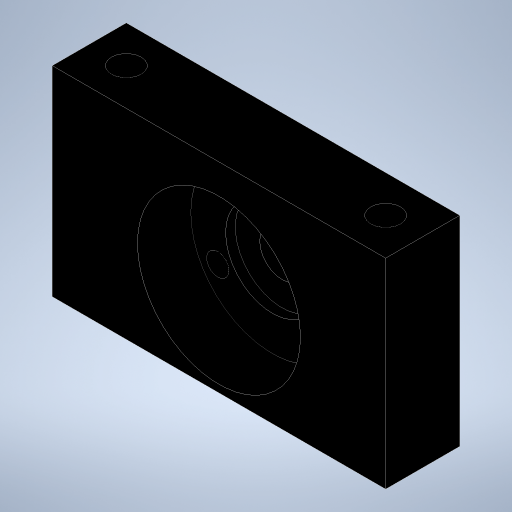
# Autodesk Inventor part: MotorBracket
Saved by Autodesk Inventor 2024 (Build 280153000, 153)
## iProperties
Created: 2023-02-23
Part Number: MotorBracket
Material: Generic
Document SubType Name: Modeling
Designer: Elias Braun
Density: 1 g/cm^3
Appearance: Default
Author: Elias Braun
Autodesk Inventor part; units mm, degrees
ref_plane "YZ Plane" through (0, 0, 0) normal (1, 0, 0) x (0, 1, 0)
ref_plane "XZ Plane" through (0, 0, 0) normal (0, 1, 0) x (-1, 0, 0)
ref_plane "XY Plane" through (0, 0, 0) normal (0, 0, 1) x (1, 0, 0)
sketch "Sketch1" plane through (0, 0, 0) normal (0, 1, 0) x (-1, 0, 0)
  line L0 (22.5, 5) -> (-22.5, 5)
  line L1 (-22.5, 5) -> (-22.5, -5)
  line L2 (-22.5, -5) -> (22.5, -5)
  line L3 (22.5, -5) -> (22.5, 5)
  line L4 (22.5, 5) -> (-22.5, -5) construction
  line L5 (-22.5, 5) -> (22.5, -5) construction
  line L6 (0, 0) -> (17.5, 0) construction
  line L7 (0, 0) -> (-17.5, 0) construction
  circle A0 centre (17.5, 0) radius 2
  circle A1 centre (-17.5, 0) radius 2
  line L8 (22.5, 5) -> (17.5, 5)
  line L9 (17.5, 5) -> (17.5, 0) construction
  dimension "d0" = 45
  dimension "d1" = 10
  dimension "d2" = 17.5
  dimension "d3" = 17.5
  dimension "d4" = 4
  dimension "d5" = 4
  constraints: 20 end point, 3 horizontal, 2 centre point, 2 coincident, 2 midpoint, 2 parallel, 1 perpendicular, 1 point on line
  measures "d0" distance of L0.start L0.end
  measures "d1" distance of L1.end L0.end
  measures "d2" distance of L6.start L6.end
  measures "d3" distance of L6.start L7.end
  measures "d4" diameter of A0
  measures "d5" diameter of A1
extrude "Extrusion1" add sketch "Sketch1" along normal blind 30
sketch "Sketch2" plane through (0, 0, 0) normal (0, -1, 0) x (1, 0, 0)
  line L0 (-22.5, -5) -> (-22.5, 5) projected
  line L1 (22.5, -5) -> (-22.5, -5) projected
  line L2 (-22.5, 5) -> (22.5, 5)
  line L3 (22.5, 5) -> (22.5, -5)
  line L4 (22.5, -5) -> (-22.5, -5)
  line L5 (-22.5, -5) -> (-22.5, 5)
  circle A0 centre (-17.5, 0) radius 2 projected
  circle A1 centre (-17.5, 0) radius 1.6
  circle A2 centre (17.5, 0) radius 2 projected
  circle A3 centre (17.5, 0) radius 1.6
  constraints: 8 end point, 2 centre point, 2 coincident, 2 parallel, 1 horizontal, 1 perpendicular
sketch "Sketch3" plane through (-22.5, 0, 5) normal (0, 0, 1) x (1, 0, 0)
  line L0 (45, 30) -> (0, 30) construction
  line L1 (0, 30) -> (45, 0) construction
  line L2 (45, 0) -> (0, 0) construction
  line L3 (45, 30) -> (0, 0) construction
  circle A0 centre (22.5, 15) radius 3
  circle A1 centre (22.5, 15) radius 7.5 construction
  circle A2 centre (22.5, 22.5) radius 1.1
  circle A3 centre (16.0048, 11.25) radius 1.1
  circle A4 centre (28.9952, 11.25) radius 1.1
  point P0 (22.5, 0)
  dimension "d9" = 15
  dimension "d8" = 6
  dimension "d10" = 2.2
  dimension "d13" = 360
  constraints: 4 centre point, 4 end point, 1 coincident, 1 midpoint, 1 vertical alignment, 9 other
  measures "d8" diameter of A0
  measures "d10" diameter of A2
extrude "Extrusion2" cut sketch "Sketch3" against normal blind 30 contours A0
sketch "Sketch4" plane through (-22.5, 0, 5) normal (0, 0, 1) x (1, 0, 0)
  line L0 (45, 0) -> (45, 30) construction
  line L1 (0, 30) -> (45, 0) construction
  line L2 (45, 30) -> (0, 30) construction
  line L3 (0, 0) -> (45, 30) construction
  circle A0 centre (22.5, 15) radius 6.3
  point P0 (22.5, 0)
  dimension "d17" = 12.6
  constraints: 4 end point, 1 centre point, 1 midpoint
  measures "d17" diameter of A0
extrude "Extrusion3" cut sketch "Sketch4" against normal blind 8.5
sketch "Sketch5" plane through (-22.5, 0, 5) normal (0, 0, 1) x (1, 0, 0)
  line L0 (0, 0) -> (0, 30) construction
  line L1 (0, 0) -> (45, 0) construction
  line L2 (0, 30) -> (45, 0) construction
  line L3 (0, 30) -> (45, 30) construction
  line L4 (45, 30) -> (0, 0) construction
  circle A0 centre (22.5, 15) radius 11
  point P0 (22.5, 0)
  dimension "d20" = 22
  constraints: 4 end point, 1 centre point, 1 midpoint
  measures "d20" diameter of A0
extrude "Extrusion4" cut sketch "Sketch5" against normal blind 7.2
extrude "Extrusion5" cut sketch "Sketch2" against normal blind 3 contours L0 L2 L3 L1
sketch "Sketch6" plane through (22.5, 30, -5) normal (0, 0, -1) x (-1, 0, 0)
  circle A0 centre (22.5, -15) radius 3 projected
  circle A1 centre (22.5, -15) radius 8.5 construction
  point P0 (22.5, -30)
  point P1 (22.5, -6.5)
  point P2 (15.1388, -19.25)
  point P3 (29.8612, -19.25)
  dimension "d25" = 17
  dimension "d28" = 360
  constraints: 2 coincident, 1 vertical alignment, 6 other
hole "Bohrung2" at (0, 15, -5) at (7.3612, 10.75, -5) at (-7.3612, 10.75, -5) at (0, 23.5, -5) direction (0, 0, 1) diameter 3 end through all
body "Solid1"
